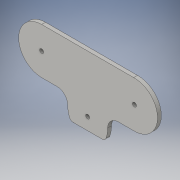
# Autodesk Inventor part: casing
Saved by Autodesk Inventor 2016 (Build 200138000, 138)
## iProperties
Created: 2019-02-22
Part Number: casing
Material: Generic
Document SubType Name: Modeling
Designer: reesem783
Density: 1 g/cm^3
Appearance: Default
Author: reesem783
Autodesk Inventor part; units mm, degrees
ref_plane "YZ Plane" through (0, 0, 0) normal (1, 0, 0) x (0, 1, 0)
ref_plane "XZ Plane" through (0, 0, 0) normal (0, 1, 0) x (-1, 0, 0)
ref_plane "XY Plane" through (0, 0, 0) normal (0, 0, 1) x (1, 0, 0)
sketch "Sketch1" plane through (0, 0, 0) normal (0, 0, 1) x (1, 0, 0)
  line L0 (0, 0) -> (76.2, 0)
  arc A0 (0, 0) -> (0, -38.1) centre (0, -19.05) ccw
  arc A1 (76.2, -38.1) -> (76.2, 0) centre (76.852, -19.05) ccw
  line L1 (76.2, -38.1) -> (63.5, -38.1)
  line L2 (0, -38.1) -> (12.7, -38.1)
  arc A2 (21.5833, -46.9837) -> (12.7, -38.1) centre (12.7, -46.9833) ccw
  arc A3 (21.5833, -46.9837) -> (22.9529, -55.026) centre (45.8763, -46.9845) ccw
  arc A4 (22.9529, -55.026) -> (25.9489, -57.15) centre (25.9489, -53.975) ccw
  arc A5 (63.5, -38.1) -> (54.6167, -46.9837) centre (63.5, -46.9833) ccw
  arc A6 (53.2471, -55.026) -> (54.6167, -46.9837) centre (30.3237, -46.9845) ccw
  arc A7 (50.2511, -57.15) -> (53.2471, -55.026) centre (50.2511, -53.975) ccw
  line L3 (25.9489, -57.15) -> (50.2511, -57.15)
  circle A8 centre (0, -19.05) radius 1.651
  circle A9 centre (76.852, -19.05) radius 1.651
  circle A10 centre (38.1, -46.9845) radius 1.651
  point P0 (23.8125, -57.15)
  dimension "d0" = 76.2
  dimension "d1" = 38.1
  dimension "d5" = 12.7
  dimension "d6" = 12.7
  dimension "d8" = 3.175
  dimension "d9" = 3.302
  dimension "d10" = 3.302
  dimension "d11" = 3.302
  constraints: 17 point on circle, 11 centre point, 8 end point, 4 tangent, 3 horizontal, 2 coincident, 1 point on line
  measures "d0" distance of L0.start L0.end
  measures "d1" distance of L0.start L2.start
  measures "d5" distance of L1.start L1.end
  measures "d6" distance of L2.start L2.end
  measures "d8" radius of A4
  measures "d9" diameter of A8
  measures "d10" diameter of A9
  measures "d11" diameter of A10
extrude "Extrusion1" add sketch "Sketch1" along normal blind 3.175
body "Solid1"
